Autodesk Inventor part; units mm, degrees
(part 2 of 2)
  dimension "d164" = 0.75
  dimension "d165" = 2
  dimension "d166" = 26
  dimension "d167" = 26
  dimension "d168" = 4
  dimension "d169" = 40
  dimension "d170" = 8
  dimension "d171" = 0.75
  dimension "d172" = 0.75
  dimension "d173" = 2
  constraints: 1200 end point, 253 vertical, 240 point on circle, 238 horizontal, 173 tangent, 120 centre point, 89 point on line, 60 equal radius, 48 parallel, 36 midpoint, 24 perpendicular, 22 collinear, 1070 other
  measures "d28" distance between parallel lines of L1 L402
  measures "d29" distance between parallel lines of L456 L0
  measures "d30" distance of point (105.988, -272.849) point (109.988, -272.849)
  measures "d31" distance of point (105.988, -312.849) point (105.988, -272.849)
  measures "d34" distance between parallel lines of L487 L486
  measures "d36" radius of A24
  measures "d37" distance between parallel lines of L491 L488
  measures "d38" distance between parallel lines of L455 L491
  measures "d39" radius of A25
  measures "d40" radius of A28
  measures "d114" distance from line of L490.start L0
  measures "d115" distance from line of L1 point (104.488, -40.525)
  measures "d116" distance of L490.start point (104.488, -208.849)
  measures "d117" distance of point (104.488, -40.525) point (104.488, -124.525)
  measures "d118" distance of point (105.988, -188.849) point (109.988, -188.849)
  measures "d119" distance of point (105.988, -228.849) point (105.988, -188.849)
  measures "d120" distance between parallel lines of L498 L497
  measures "d121" radius of A32
  measures "d122" radius of A33
  measures "d123" radius of A36
  measures "d124" distance of point (105.988, -104.525) point (109.988, -104.525)
  measures "d125" distance of point (105.988, -144.525) point (105.988, -104.525)
  measures "d126" distance between parallel lines of L507 L506
  measures "d127" radius of A40
  measures "d128" radius of A41
  measures "d129" radius of A44
  measures "d130" distance of point (105.988, -20.525) point (109.988, -20.525)
  measures "d131" distance of point (105.988, -60.525) point (105.988, -20.525)
  measures "d132" distance between parallel lines of L516 L515
  measures "d133" radius of A48
  measures "d134" radius of A49
  measures "d135" radius of A52
  measures "d142" distance of point (-1.5, -312.849) point (-5.5, -312.849)
  measures "d143" distance of point (-1.5, -272.849) point (-1.5, -312.849)
  measures "d144" distance between parallel lines of L535 L528
  measures "d145" radius of A58
  measures "d146" radius of A56
  measures "d147" radius of A57
  measures "d148" distance of point (-1.5, -228.849) point (-5.5, -228.849)
  measures "d149" distance of point (-1.5, -188.849) point (-1.5, -228.849)
  measures "d150" distance between parallel lines of L541 L545
  measures "d151" radius of A66
  measures "d152" radius of A67
  measures "d153" radius of A70
  measures "d154" distance of point (-1.5, -144.525) point (-5.5, -144.525)
  measures "d155" distance of point (-1.5, -104.525) point (-1.5, -144.525)
  measures "d156" distance between parallel lines of L550 L554
  measures "d157" radius of A74
  measures "d158" radius of A75
  measures "d159" radius of A78
  measures "d160" distance of point (-1.5, -60.525) point (-5.5, -60.525)
  measures "d161" distance of point (-1.5, -20.525) point (-1.5, -60.525)
  measures "d162" distance between parallel lines of L559 L563
  measures "d163" radius of A82
  measures "d164" radius of A83
  measures "d165" radius of A86
  measures "d166" distance from line of point (78.488, 1.475) L523
  measures "d167" distance from line of L493 point (26, 1.475)
  measures "d168" distance of point (58.488, 2.975) point (58.488, 6.975)
  measures "d169" distance of point (98.488, 2.975) point (58.488, 2.975)
  measures "d170" distance between parallel lines of L571 L564
  measures "d171" radius of A90
  measures "d172" radius of A88
  measures "d173" radius of A89
extrude "拉伸1" add sketch "草图1" along normal blind 1.5
fillet "圆角1" radius 2 4 edges at (-104.4878, 0.75, 1.4754) (0, 0.75, 1.4754) (0, 0.75, -334.8489) (-104.4878, 0.75, -334.8489)
